Autodesk Fusion 360 part; units mm, degrees
note: some values were not read from the file. Set by a fixed rule: which sketch regions a step uses.
(part 5 of 59)
  spline S22 degree 5 poles (22.1904, 31.2406) (22.1905, 31.2407) (22.1907, 31.2408) (22.1909, 31.241) (22.1913, 31.2414) (22.1919, 31.2419) (22.1925, 31.2424) (22.1933, 31.2431) (22.1941, 31.2438) (22.195, 31.2446) (22.196, 31.2455) (22.197, 31.2464) (22.1982, 31.2474) (22.1994, 31.2485) (22.2007, 31.2497) (22.202, 31.2509) (22.2035, 31.2522) (22.205, 31.2536) (22.2066, 31.255) (22.2082, 31.2565) (22.2099, 31.2581) (22.2117, 31.2597) (22.2136, 31.2615) (22.2155, 31.2632) (22.2175, 31.2651) (22.2195, 31.267) (22.2216, 31.269) (22.2238, 31.271) (22.226, 31.2732) (22.2283, 31.2753) (22.2307, 31.2776) (22.2331, 31.2799) (22.2355, 31.2823) (22.238, 31.2847) (22.2406, 31.2872) (22.2433, 31.2897) (22.2459, 31.2924) (22.2487, 31.2951) (22.2515, 31.2978) (22.2543, 31.3006) (22.2572, 31.3035) (22.2602, 31.3064) (22.2632, 31.3094) (22.2662, 31.3124) (22.2693, 31.3156) (22.2725, 31.3187) (22.2757, 31.322) (22.2789, 31.3252) (22.2822, 31.3286) (22.2855, 31.332) (22.2889, 31.3355) (22.2923, 31.339) (22.2958, 31.3426) (22.2993, 31.3462) (22.3029, 31.3499) (22.3065, 31.3536) (22.3101, 31.3574) (22.3138, 31.3613) (22.3175, 31.3652) (22.3212, 31.3692) (22.325, 31.3732) (22.3289, 31.3773) (22.3328, 31.3814) (22.3367, 31.3856) (22.3406, 31.3899) (22.3446, 31.3942) (22.3486, 31.3986) (22.3527, 31.403) (22.3568, 31.4074) (22.3609, 31.4119) (22.3651, 31.4165) (22.3693, 31.4211) (22.3736, 31.4258) (22.3778, 31.4306) (22.3821, 31.4353) (22.3865, 31.4402) (22.3909, 31.4451) (22.3953, 31.45) (22.3997, 31.455) (22.4042, 31.46) (22.4087, 31.4651) (22.4132, 31.4703) (22.4177, 31.4755) (22.4223, 31.4807) (22.427, 31.486) (22.4316, 31.4914) (22.4363, 31.4968) (22.441, 31.5022) (22.4457, 31.5077) (22.4505, 31.5133) (22.4553, 31.5189) (22.4601, 31.5246) (22.4649, 31.5303) (22.4698, 31.536) (22.4747, 31.5418) (22.4796, 31.5477) (22.4846, 31.5536) (22.4895, 31.5595) (22.4945, 31.5655) (22.4996, 31.5715) (22.5046, 31.5776) (22.5097, 31.5838) (22.5148, 31.59) (22.5199, 31.5962) (22.525, 31.6025) (22.5302, 31.6088) (22.5354, 31.6152) (22.5406, 31.6216) (22.5458, 31.6281) (22.5511, 31.6346) (22.5564, 31.6412) (22.5617, 31.6478) (22.567, 31.6544) (22.5723, 31.6611) (22.5777, 31.6679) (22.583, 31.6747) (22.5884, 31.6815) (22.5939, 31.6884) (22.5993, 31.6954) (22.6048, 31.7024) (22.6102, 31.7094) (22.6157, 31.7165) (22.6212, 31.7236) (22.6268, 31.7307) (22.6323, 31.7379) (22.6379, 31.7452) (22.6435, 31.7525) (22.6491, 31.7598) (22.6547, 31.7672) (22.6603, 31.7747) (22.666, 31.7821) (22.6716, 31.7897) (22.6773, 31.7972) (22.683, 31.8048) (22.6887, 31.8125) (22.6945, 31.8202) (22.7002, 31.8279) (22.706, 31.8357) (22.7118, 31.8436) (22.7175, 31.8514) (22.7233, 31.8593) (22.7292, 31.8673) (22.735, 31.8753) (22.7408, 31.8834) (22.7467, 31.8914) (22.7526, 31.8996) (22.7585, 31.9078) (22.7644, 31.916) (22.7703, 31.9242) (22.7762, 31.9325) (22.7822, 31.9409) (22.7881, 31.9493) (22.7941, 31.9577) (22.8, 31.9662) (22.806, 31.9747) (22.812, 31.9832) (22.818, 31.9918) (22.8241, 32.0005) (22.8301, 32.0091) (22.8361, 32.0179) (22.8422, 32.0266) (22.8483, 32.0354) (22.8543, 32.0443) (22.8604, 32.0532) (22.8665, 32.0621) (22.8726, 32.0711) (22.8787, 32.0801) (22.8849, 32.0891) (22.891, 32.0982) (22.8971, 32.1073) (22.9033, 32.1165) (22.9095, 32.1257) (22.9156, 32.135) (22.9218, 32.1443) (22.928, 32.1536) (22.9342, 32.163) (22.9404, 32.1724) (22.9466, 32.1818) (22.9528, 32.1913) (22.9591, 32.2009) (22.9653, 32.2104) (22.9715, 32.22) (22.9778, 32.2297) (22.984, 32.2394) (22.9903, 32.2491) (22.9966, 32.2589) (23.0029, 32.2687) (23.0091, 32.2785) (23.0154, 32.2884) (23.0217, 32.2984) (23.028, 32.3083) (23.0343, 32.3183) (23.0406, 32.3284) (23.047, 32.3384) (23.0533, 32.3486) (23.0596, 32.3587) (23.066, 32.3689) (23.0723, 32.3791) (23.0786, 32.3894) (23.085, 32.3997) (23.0914, 32.4101) (23.0977, 32.4205) (23.1041, 32.4309) (23.1104, 32.4413) (23.1168, 32.4518) (23.1232, 32.4624) (23.1296, 32.473) (23.136, 32.4836) (23.1423, 32.4942) (23.1487, 32.5049) (23.1551, 32.5156) (23.1615, 32.5264) (23.1679, 32.5372) (23.1743, 32.548) (23.1807, 32.5589) (23.1872, 32.5698) (23.1936, 32.5808) (23.2, 32.5917) (23.2064, 32.6028) (23.2128, 32.6138) (23.2193, 32.6249) (23.2257, 32.636) (23.2321, 32.6472) (23.2385, 32.6584) (23.245, 32.6697) (23.2514, 32.6809) (23.2578, 32.6922) (23.2643, 32.7036) (23.2707, 32.715) (23.2771, 32.7264) (23.2836, 32.7379) (23.29, 32.7493) (23.2965, 32.7609) (23.3029, 32.7724) (23.3094, 32.784) (23.3158, 32.7957) (23.3222, 32.8073) (23.3287, 32.819) (23.3351, 32.8308) (23.3416, 32.8426) (23.348, 32.8544) (23.3532, 32.8639) (23.3571, 32.871) (23.3596, 32.8757) (23.3609, 32.8781) knots 0 0 0 0 0 0 0.00416667 0.00833333 0.0125 0.01666667 0.02083333 0.025 0.02916667 0.03333333 0.0375 0.04166667 0.04583333 0.05 0.05416667 0.05833333 0.0625 0.06666667 0.07083333 0.075 0.07916667 0.08333333 0.0875 0.09166667 0.09583333 0.1 0.10416667 0.10833333 0.1125 0.11666667 0.12083333 0.125 0.12916667 0.13333333 0.1375 0.14166667 0.14583333 0.15 0.15416667 0.15833333 0.1625 0.16666667 0.17083333 0.175 0.17916667 0.18333333 0.1875 0.19166667 0.19583333 0.2 0.20416667 0.20833333 0.2125 0.21666667 0.22083333 0.225 0.22916667 0.23333333 0.2375 0.24166667 0.24583333 0.25 0.25416667 0.25833333 0.2625 0.26666667 0.27083333 0.275 0.27916667 0.28333333 0.2875 0.29166667 0.29583333 0.3 0.30416667 0.30833333 0.3125 0.31666667 0.32083333 0.325 0.32916667 0.33333333 0.3375 0.34166667 0.34583333 0.35 0.35416667 0.35833333 0.3625 0.36666667 0.37083333 0.375 0.37916667 0.38333333 0.3875 0.39166667 0.39583333 0.4 0.40416667 0.40833333 0.4125 0.41666667 0.42083333 0.425 0.42916667 0.43333333 0.4375 0.44166667 0.44583333 0.45 0.45416667 0.45833333 0.4625 0.46666667 0.47083333 0.475 0.47916667 0.48333333 0.4875 0.49166667 0.49583333 0.5 0.50416667 0.50833333 0.5125 0.51666667 0.52083333 0.525 0.52916667 0.53333333 0.5375 0.54166667 0.54583333 0.55 0.55416667 0.55833333 0.5625 0.56666667 0.57083333 0.575 0.57916667 0.58333333 0.5875 0.59166667 0.59583333 0.6 0.60416667 0.60833333 0.6125 0.61666667 0.62083333 0.625 0.62916667 0.63333333 0.6375 0.64166667 0.64583333 0.65 0.65416667 0.65833333 0.6625 0.66666667 0.67083333 0.675 0.67916667 0.68333333 0.6875 0.69166667 0.69583333 0.7 0.70416667 0.70833333 0.7125 0.71666667 0.72083333 0.725 0.72916667 0.73333333 0.7375 0.74166667 0.74583333 0.75 0.75416667 0.75833333 0.7625 0.76666667 0.77083333 0.775 0.77916667 0.78333333 0.7875 0.79166667 0.79583333 0.8 0.80416667 0.80833333 0.8125 0.81666667 0.82083333 0.825 0.82916667 0.83333333 0.8375 0.84166667 0.84583333 0.85 0.85416667 0.85833333 0.8625 0.86666667 0.87083333 0.875 0.87916667 0.88333333 0.8875 0.89166667 0.89583333 0.9 0.90416667 0.90833333 0.9125 0.91666667 0.92083333 0.925 0.92916667 0.93333333 0.9375 0.94166667 0.94583333 0.95 0.95416667 0.95833333 0.9625 0.96666667 0.97083333 0.975 0.97916667 0.98333333 0.9875 0.99166667 0.99583333 1 1 1 1 1 1
  line L72 (-28.5878, 17.6346) -> (-28.587, 17.6345)
  line L73 (-15.1575, -11.9297) -> (-15.3128, -12.1799)
  line L74 (-27.918, 19.3665) -> (-28.2039, 19.4368)
  spline S23 degree 5 poles (-29.3284, 2.4579) (-29.3257, 2.4578) (-29.3203, 2.4577) (-29.3122, 2.4575) (-29.3014, 2.4572) (-29.288, 2.4569) (-29.2745, 2.4566) (-29.2612, 2.4563) (-29.2478, 2.456) (-29.2345, 2.4558) (-29.2212, 2.4555) (-29.2079, 2.4553) (-29.1947, 2.4551) (-29.1815, 2.4549) (-29.1683, 2.4547) (-29.1551, 2.4546) (-29.142, 2.4545) (-29.129, 2.4543) (-29.1159, 2.4542) (-29.1029, 2.4542) (-29.0899, 2.4541) (-29.077, 2.454) (-29.0641, 2.454) (-29.0512, 2.454) (-29.0383, 2.454) (-29.0255, 2.454) (-29.0127, 2.454) (-29, 2.4541) (-28.9872, 2.4542) (-28.9745, 2.4542) (-28.9619, 2.4543) (-28.9493, 2.4544) (-28.9367, 2.4546) (-28.9241, 2.4547) (-28.9116, 2.4549) (-28.8991, 2.4551) (-28.8867, 2.4552) (-28.8743, 2.4555) (-28.8619, 2.4557) (-28.8495, 2.4559) (-28.8372, 2.4562) (-28.8249, 2.4564) (-28.8127, 2.4567) (-28.8005, 2.457) (-28.7883, 2.4573) (-28.7762, 2.4577) (-28.7641, 2.458) (-28.752, 2.4584) (-28.74, 2.4588) (-28.728, 2.4591) (-28.716, 2.4595) (-28.7041, 2.46) (-28.6922, 2.4604) (-28.6803, 2.4608) (-28.6685, 2.4613) (-28.6567, 2.4618) (-28.645, 2.4623) (-28.6333, 2.4628) (-28.6216, 2.4633) (-28.61, 2.4638) (-28.5984, 2.4644) (-28.5868, 2.4649) (-28.5753, 2.4655) (-28.5638, 2.4661) (-28.5524, 2.4667) (-28.541, 2.4673) (-28.5296, 2.4679) (-28.5183, 2.4686) (-28.507, 2.4692) (-28.4957, 2.4699) (-28.4845, 2.4706) (-28.4733, 2.4713) (-28.4622, 2.472) (-28.4511, 2.4727) (-28.44, 2.4734) (-28.429, 2.4742) (-28.4181, 2.4749) (-28.4071, 2.4757) (-28.3962, 2.4765) (-28.3854, 2.4773) (-28.3745, 2.4781) (-28.3638, 2.4789) (-28.353, 2.4797) (-28.3423, 2.4805) (-28.3317, 2.4814) (-28.321, 2.4823) (-28.3105, 2.4831) (-28.2999, 2.484) (-28.2894, 2.4849) (-28.279, 2.4858) (-28.2686, 2.4867) (-28.2582, 2.4877) (-28.2479, 2.4886) (-28.2376, 2.4896) (-28.2274, 2.4905) (-28.2172, 2.4915) (-28.207, 2.4925) (-28.1969, 2.4935) (-28.1868, 2.4945) (-28.1768, 2.4955) (-28.1668, 2.4965) (-28.1569, 2.4975) (-28.147, 2.4986) (-28.1372, 2.4996) (-28.1274, 2.5007) (-28.1176, 2.5017) (-28.1079, 2.5028) (-28.0982, 2.5039) (-28.0886, 2.505) (-28.079, 2.5061) (-28.0695, 2.5072) (-28.06, 2.5084) (-28.0506, 2.5095) (-28.0412, 2.5106) (-28.0318, 2.5118) (-28.0225, 2.5129) (-28.0133, 2.5141) (-28.004, 2.5153) (-27.9949, 2.5164) (-27.9858, 2.5176) (-27.9767, 2.5188) (-27.9677, 2.52) (-27.9587, 2.5212) (-27.9498, 2.5224) (-27.9409, 2.5237) (-27.9321, 2.5249) (-27.9233, 2.5261) (-27.9146, 2.5274) (-27.9059, 2.5286) (-27.8973, 2.5299) (-27.8887, 2.5311) (-27.8802, 2.5324) (-27.8717, 2.5336) (-27.8633, 2.5349) (-27.8549, 2.5362) (-27.8466, 2.5375) (-27.8383, 2.5388) (-27.8301, 2.5401) (-27.8219, 2.5414) (-27.8138, 2.5427) (-27.8057, 2.544) (-27.7977, 2.5453) (-27.7898, 2.5466) (-27.7819, 2.5479) (-27.774, 2.5492) (-27.7662, 2.5506) (-27.7585, 2.5519) (-27.7508, 2.5532) (-27.7431, 2.5546) (-27.7356, 2.5559) (-27.728, 2.5572) (-27.7206, 2.5586) (-27.7132, 2.5599) (-27.7058, 2.5613) (-27.6985, 2.5626) (-27.6912, 2.564) (-27.6841, 2.5653) (-27.6769, 2.5667) (-27.6698, 2.568) (-27.6628, 2.5694) (-27.6559, 2.5707) (-27.649, 2.5721) (-27.6421, 2.5734) (-27.6353, 2.5748) (-27.6286, 2.5761) (-27.622, 2.5775) (-27.6154, 2.5788) (-27.6088, 2.5801) (-27.6023, 2.5815) (-27.5959, 2.5828) (-27.5896, 2.5842) (-27.5833, 2.5855) (-27.577, 2.5868) (-27.5709, 2.5882) (-27.5647, 2.5895) (-27.5587, 2.5908) (-27.5527, 2.5921) (-27.5468, 2.5935) (-27.5409, 2.5948) (-27.5352, 2.5961) (-27.5294, 2.5974) (-27.5238, 2.5987) (-27.5182, 2.6) (-27.5127, 2.6013) (-27.5072, 2.6026) (-27.5018, 2.6038) (-27.4965, 2.6051) (-27.4912, 2.6064) (-27.4861, 2.6076) (-27.481, 2.6089) (-27.4759, 2.6101) (-27.4709, 2.6113) (-27.466, 2.6126) (-27.4612, 2.6138) (-27.4564, 2.615) (-27.4517, 2.6162) (-27.4471, 2.6173) (-27.4426, 2.6185) (-27.4381, 2.6197) (-27.4337, 2.6208) (-27.4294, 2.622) (-27.4252, 2.6231) (-27.421, 2.6242) (-27.4169, 2.6253) (-27.4129, 2.6264) (-27.409, 2.6275) (-27.4051, 2.6285) (-27.4013, 2.6296) (-27.3976, 2.6306) (-27.394, 2.6316) (-27.3905, 2.6326) (-27.387, 2.6336) (-27.3837, 2.6346) (-27.3804, 2.6355) (-27.3772, 2.6365) (-27.3741, 2.6374) (-27.371, 2.6383) (-27.3681, 2.6392) (-27.3652, 2.64) (-27.3625, 2.6409) (-27.3598, 2.6417) (-27.3572, 2.6425) (-27.3547, 2.6432) (-27.3523, 2.644) (-27.3499, 2.6447) (-27.3477, 2.6454) (-27.3456, 2.6461) (-27.3435, 2.6467) (-27.3416, 2.6473) (-27.3398, 2.6479) (-27.338, 2.6485) (-27.3364, 2.649) (-27.3348, 2.6495) (-27.3334, 2.65) (-27.332, 2.6505) (-27.3308, 2.6509) (-27.3296, 2.6513) (-27.3286, 2.6516) (-27.3277, 2.6519) (-27.3269, 2.6522) (-27.3262, 2.6525) (-27.3257, 2.6526) (-27.3254, 2.6527) (-27.3252, 2.6528) (-27.3251, 2.6528) knots -1 -1 -1 -1 -1 -1 -0.99583333 -0.99166667 -0.9875 -0.98333333 -0.97916667 -0.975 -0.97083333 -0.96666667 -0.9625 -0.95833333 -0.95416667 -0.95 -0.94583333 -0.94166667 -0.9375 -0.93333333 -0.92916667 -0.925 -0.92083333 -0.91666667 -0.9125 -0.90833333 -0.90416667 -0.9 -0.89583333 -0.89166667 -0.8875 -0.88333333 -0.87916667 -0.875 -0.87083333 -0.86666667 -0.8625 -0.85833333 -0.85416667 -0.85 -0.84583333 -0.84166667 -0.8375 -0.83333333 -0.82916667 -0.825 -0.82083333 -0.81666667 -0.8125 -0.80833333 -0.80416667 -0.8 -0.79583333 -0.79166667 -0.7875 -0.78333333 -0.77916667 -0.775 -0.77083333 -0.76666667 -0.7625 -0.75833333 -0.75416667 -0.75 -0.74583333 -0.74166667 -0.7375 -0.73333333 -0.72916667 -0.725 -0.72083333 -0.71666667 -0.7125 -0.70833333 -0.70416667 -0.7 -0.69583333 -0.69166667 -0.6875 -0.68333333 -0.67916667 -0.675 -0.67083333 -0.66666667 -0.6625 -0.65833333 -0.65416667 -0.65 -0.64583333 -0.64166667 -0.6375 -0.63333333 -0.62916667 -0.625 -0.62083333 -0.61666667 -0.6125 -0.60833333 -0.60416667 -0.6 -0.59583333 -0.59166667 -0.5875 -0.58333333 -0.57916667 -0.575 -0.57083333 -0.56666667 -0.5625 -0.55833333 -0.55416667 -0.55 -0.54583333 -0.54166667 -0.5375 -0.53333333 -0.52916667 -0.525 -0.52083333 -0.51666667 -0.5125 -0.50833333 -0.50416667 -0.5 -0.49583333 -0.49166667 -0.4875 -0.48333333 -0.47916667 -0.475 -0.47083333 -0.46666667 -0.4625 -0.45833333 -0.45416667 -0.45 -0.44583333 -0.44166667 -0.4375 -0.43333333 -0.42916667 -0.425 -0.42083333 -0.41666667 -0.4125 -0.40833333 -0.40416667 -0.4 -0.39583333 -0.39166667 -0.3875 -0.38333333 -0.37916667 -0.375 -0.37083333 -0.36666667 -0.3625 -0.35833333 -0.35416667 -0.35 -0.34583333 -0.34166667 -0.3375 -0.33333333 -0.32916667 -0.325 -0.32083333 -0.31666667 -0.3125 -0.30833333 -0.30416667 -0.3 -0.29583333 -0.29166667 -0.2875 -0.28333333 -0.27916667 -0.275 -0.27083333 -0.26666667 -0.2625 -0.25833333 -0.25416667 -0.25 -0.24583333 -0.24166667 -0.2375 -0.23333333 -0.22916667 -0.225 -0.22083333 -0.21666667 -0.2125 -0.20833333 -0.20416667 -0.2 -0.19583333 -0.19166667 -0.1875 -0.18333333 -0.17916667 -0.175 -0.17083333 -0.16666667 -0.1625 -0.15833333 -0.15416667 -0.15 -0.14583333 -0.14166667 -0.1375 -0.13333333 -0.12916667 -0.125 -0.12083333 -0.11666667 -0.1125 -0.10833333 -0.10416667 -0.1 -0.09583333 -0.09166667 -0.0875 -0.08333333 -0.07916667 -0.075 -0.07083333 -0.06666667 -0.0625 -0.05833333 -0.05416667 -0.05 -0.04583333 -0.04166667 -0.0375 -0.03333333 -0.02916667 -0.025 -0.02083333 -0.01666667 -0.0125 -0.00833333 -0.00416667 0 0 0 0 0 0
  line L75 (-25.6012, -1.2171) -> (-25.6019, -1.2175)
  line L76 (-26.1461, -0.1495) -> (-26.1453, -0.1491)
  arc A31 (-27.6109, 20.5125) -> (-27.918, 19.3665) centre (0, 12.5) ccw
  arc A32 (-30.2174, 19.4214) -> (-30.4202, 18.4675) centre (0, 12.5) ccw
  spline S24 degree 5 poles (-30.4202, 18.4675) (-30.4179, 18.4661) (-30.4133, 18.4633) (-30.4064, 18.459) (-30.3972, 18.4534) (-30.3857, 18.4464) (-30.3742, 18.4394) (-30.3628, 18.4325) (-30.3513, 18.4255) (-30.3399, 18.4187) (-30.3285, 18.4118) (-30.3171, 18.405) (-30.3058, 18.3982) (-30.2944, 18.3914) (-30.2831, 18.3847) (-30.2718, 18.378) (-30.2605, 18.3713) (-30.2492, 18.3647) (-30.238, 18.3581) (-30.2268, 18.3515) (-30.2156, 18.3449) (-30.2044, 18.3384) (-30.1932, 18.3319) (-30.1821, 18.3255) (-30.1709, 18.3191) (-30.1598, 18.3127) (-30.1487, 18.3063) (-30.1377, 18.3) (-30.1266, 18.2937) (-30.1156, 18.2874) (-30.1046, 18.2811) (-30.0936, 18.2749) (-30.0826, 18.2688) (-30.0717, 18.2626) (-30.0608, 18.2565) (-30.0499, 18.2504) (-30.039, 18.2443) (-30.0281, 18.2383) (-30.0173, 18.2323) (-30.0065, 18.2263) (-29.9957, 18.2204) (-29.9849, 18.2145) (-29.9742, 18.2086) (-29.9634, 18.2028) (-29.9527, 18.197) (-29.9421, 18.1912) (-29.9314, 18.1854) (-29.9208, 18.1797) (-29.9102, 18.174) (-29.8996, 18.1683) (-29.889, 18.1627) (-29.8785, 18.1571) (-29.868, 18.1515) (-29.8575, 18.146) (-29.847, 18.1405) (-29.8366, 18.135) (-29.8262, 18.1296) (-29.8158, 18.1242) (-29.8054, 18.1188) (-29.7951, 18.1134) (-29.7847, 18.1081) (-29.7745, 18.1028) (-29.7642, 18.0975) (-29.754, 18.0923) (-29.7437, 18.0871) (-29.7336, 18.0819) (-29.7234, 18.0768) (-29.7133, 18.0717) (-29.7032, 18.0666) (-29.6931, 18.0615) (-29.683, 18.0565) (-29.673, 18.0515) (-29.663, 18.0466) (-29.653, 18.0416) (-29.6431, 18.0367) (-29.6332, 18.0319) (-29.6233, 18.027) (-29.6134, 18.0222) (-29.6036, 18.0175) (-29.5938, 18.0127) (-29.584, 18.008) (-29.5743, 18.0033) (-29.5646, 17.9987) (-29.5549, 17.994) (-29.5452, 17.9895) (-29.5356, 17.9849) (-29.526, 17.9804) (-29.5165, 17.9759) (-29.5069, 17.9714) (-29.4974, 17.967) (-29.4879, 17.9625) (-29.4785, 17.9582) (-29.4691, 17.9538) (-29.4597, 17.9495) (-29.4504, 17.9452) (-29.441, 17.941) (-29.4318, 17.9367) (-29.4225, 17.9325) (-29.4133, 17.9284) (-29.4041, 17.9242) (-29.395, 17.9201) (-29.3858, 17.9161) (-29.3767, 17.912) (-29.3677, 17.908) (-29.3587, 17.904) (-29.3497, 17.9001) (-29.3407, 17.8961) (-29.3318, 17.8922) (-29.3229, 17.8884) (-29.3141, 17.8846) (-29.3053, 17.8807) (-29.2965, 17.877) (-29.2878, 17.8732) (-29.279, 17.8695) (-29.2704, 17.8658) (-29.2617, 17.8622) (-29.2531, 17.8586) (-29.2446, 17.855) (-29.2361, 17.8514) (-29.2276, 17.8479) (-29.2191, 17.8444) (-29.2107, 17.8409) (-29.2023, 17.8375) (-29.194, 17.8341) (-29.1857, 17.8307) (-29.1775, 17.8273) (-29.1692, 17.824) (-29.1611, 17.8207) (-29.1529, 17.8175) (-29.1448, 17.8143) (-29.1368, 17.8111) (-29.1288, 17.8079) (-29.1208, 17.8047) (-29.1129, 17.8016) (-29.105, 17.7986) (-29.0971, 17.7955) (-29.0893, 17.7925) (-29.0815, 17.7895) (-29.0738, 17.7865) (-29.0661, 17.7836) (-29.0585, 17.7807) (-29.0509, 17.7778) (-29.0433, 17.775) (-29.0358, 17.7722) (-29.0284, 17.7694) (-29.021, 17.7666) (-29.0136, 17.7639) (-29.0063, 17.7612) (-28.999, 17.7586) (-28.9918, 17.7559) (-28.9846, 17.7533) (-28.9774, 17.7508) (-28.9703, 17.7482) (-28.9633, 17.7457) (-28.9563, 17.7432) (-28.9493, 17.7408) (-28.9424, 17.7383) (-28.9356, 17.7359) (-28.9288, 17.7336) (-28.922, 17.7312) (-28.9153, 17.7289) (-28.9087, 17.7266) (-28.9021, 17.7244) (-28.8955, 17.7222) (-28.889, 17.72) (-28.8826, 17.7178) (-28.8762, 17.7157) (-28.8699, 17.7136) (-28.8636, 17.7115) (-28.8573, 17.7094) (-28.8512, 17.7074) (-28.8451, 17.7054) (-28.839, 17.7035) (-28.833, 17.7015) (-28.827, 17.6996) (-28.8211, 17.6978) (-28.8153, 17.6959) (-28.8095, 17.6941) (-28.8038, 17.6923) (-28.7981, 17.6905) (-28.7925, 17.6888) (-28.7869, 17.6871) (-28.7815, 17.6854) (-28.776, 17.6838) (-28.7707, 17.6822) (-28.7654, 17.6806) (-28.7601, 17.679) (-28.7549, 17.6775) (-28.7498, 17.676) (-28.7448, 17.6745) (-28.7398, 17.673) (-28.7349, 17.6716) (-28.73, 17.6702) (-28.7252, 17.6689) (-28.7205, 17.6675) (-28.7158, 17.6662) (-28.7112, 17.6649) (-28.7067, 17.6637) (-28.7023, 17.6625) (-28.6979, 17.6613) (-28.6936, 17.6601) (-28.6893, 17.6589) (-28.6852, 17.6578) (-28.6811, 17.6567) (-28.6771, 17.6557) (-28.6731, 17.6546) (-28.6693, 17.6536) (-28.6655, 17.6527) (-28.6617, 17.6517) (-28.6581, 17.6508) (-28.6545, 17.6499) (-28.6511, 17.649) (-28.6477, 17.6481) (-28.6443, 17.6473) (-28.6411, 17.6465) (-28.6379, 17.6458) (-28.6349, 17.645) (-28.6319, 17.6443) (-28.629, 17.6436) (-28.6262, 17.643) (-28.6234, 17.6423) (-28.6208, 17.6417) (-28.6182, 17.6411) (-28.6158, 17.6406) (-28.6134, 17.64) (-28.6111, 17.6395) (-28.6089, 17.639) (-28.6069, 17.6386) (-28.6049, 17.6381) (-28.603, 17.6377) (-28.6012, 17.6374) (-28.5995, 17.637) (-28.5979, 17.6367) (-28.5964, 17.6363) (-28.595, 17.6361) (-28.5937, 17.6358) (-28.5925, 17.6356) (-28.5915, 17.6354) (-28.5905, 17.6352) (-28.5896, 17.635) (-28.5889, 17.6349) (-28.5884, 17.6348) (-28.5881, 17.6347) (-28.5879, 17.6347) (-28.5878, 17.6346) knots -1 -1 -1 -1 -1 -1 -0.99583333 -0.99166667 -0.9875 -0.98333333 -0.97916667 -0.975 -0.97083333 -0.96666667 -0.9625 -0.95833333 -0.95416667 -0.95 -0.94583333 -0.94166667 -0.9375 -0.93333333 -0.92916667 -0.925 -0.92083333 -0.91666667 -0.9125 -0.90833333 -0.90416667 -0.9 -0.89583333 -0.89166667 -0.8875 -0.88333333 -0.87916667 -0.875 -0.87083333 -0.86666667 -0.8625 -0.85833333 -0.85416667 -0.85 -0.84583333 -0.84166667 -0.8375 -0.83333333 -0.82916667 -0.825 -0.82083333 -0.81666667 -0.8125 -0.80833333 -0.80416667 -0.8 -0.79583333 -0.79166667 -0.7875 -0.78333333 -0.77916667 -0.775 -0.77083333 -0.76666667 -0.7625 -0.75833333 -0.75416667 -0.75 -0.74583333 -0.74166667 -0.7375 -0.73333333 -0.72916667 -0.725 -0.72083333 -0.71666667 -0.7125 -0.70833333 -0.70416667 -0.7 -0.69583333 -0.69166667 -0.6875 -0.68333333 -0.67916667 -0.675 -0.67083333 -0.66666667 -0.6625 -0.65833333 -0.65416667 -0.65 -0.64583333 -0.64166667 -0.6375 -0.63333333 -0.62916667 -0.625 -0.62083333 -0.61666667 -0.6125 -0.60833333 -0.60416667 -0.6 -0.59583333 -0.59166667 -0.5875 -0.58333333 -0.57916667 -0.575 -0.57083333 -0.56666667 -0.5625 -0.55833333 -0.55416667 -0.55 -0.54583333 -0.54166667 -0.5375 -0.53333333 -0.52916667 -0.525 -0.52083333 -0.51666667 -0.5125 -0.50833333 -0.50416667 -0.5 -0.49583333 -0.49166667 -0.4875 -0.48333333 -0.47916667 -0.475 -0.47083333 -0.46666667 -0.4625 -0.45833333 -0.45416667 -0.45 -0.44583333 -0.44166667 -0.4375 -0.43333333 -0.42916667 -0.425 -0.42083333 -0.41666667 -0.4125 -0.40833333 -0.40416667 -0.4 -0.39583333 -0.39166667 -0.3875 -0.38333333 -0.37916667 -0.375 -0.37083333 -0.36666667 -0.3625 -0.35833333 -0.35416667 -0.35 -0.34583333 -0.34166667 -0.3375 -0.33333333 -0.32916667 -0.325 -0.32083333 -0.31666667 -0.3125 -0.30833333 -0.30416667 -0.3 -0.29583333 -0.29166667 -0.2875 -0.28333333 -0.27916667 -0.275 -0.27083333 -0.26666667 -0.2625 -0.25833333 -0.25416667 -0.25 -0.24583333 -0.24166667 -0.2375 -0.23333333 -0.22916667 -0.225 -0.22083333 -0.21666667 -0.2125 -0.20833333 -0.20416667 -0.2 -0.19583333 -0.19166667 -0.1875 -0.18333333 -0.17916667 -0.175 -0.17083333 -0.16666667 -0.1625 -0.15833333 -0.15416667 -0.15 -0.14583333 -0.14166667 -0.1375 -0.13333333 -0.12916667 -0.125 -0.12083333 -0.11666667 -0.1125 -0.10833333 -0.10416667 -0.1 -0.09583333 -0.09166667 -0.0875 -0.08333333 -0.07916667 -0.075 -0.07083333 -0.06666667 -0.0625 -0.05833333 -0.05416667 -0.05 -0.04583333 -0.04166667 -0.0375 -0.03333333 -0.02916667 -0.025 -0.02083333 -0.01666667 -0.0125 -0.00833333 -0.00416667 0 0 0 0 0 0
  arc A33 (-28.2972, 17.5824) -> (-28.4828, 16.4106) centre (0, 12.5) ccw
  line L77 (-28.7753, 8.5492) -> (-28.7745, 8.5493)
  arc A34 (-28.5147, 0.3382) -> (-28.1181, -0.5527) centre (0, 12.5) ccw
  line L78 (-24.6799, -2.8128) -> (-24.4297, -2.6575)
  line L79 (-28.7745, 8.5493) -> (-28.4828, 8.5894)
  line L80 (-29.0307, 11.5787) -> (-29.0298, 11.5787)
  line L81 (-21.9649, -6.0501) -> (-22.1898, -6.2401)
  line L82 (-28.9671, 10.3818) -> (-28.9679, 10.3817)
  arc A35 (-27.0873, -2.5758) -> (-26.5997, -3.4204) centre (0, 12.5) ccw
  spline S25 degree 5 poles (-15.3132, -12.1806) (-15.3132, -12.1807) (-15.3133, -12.1809) (-15.3135, -12.1812) (-15.3138, -12.1816) (-15.3142, -12.1822) (-15.3146, -12.183) (-15.3151, -12.1838) (-15.3157, -12.1848) (-15.3163, -12.1858) (-15.3169, -12.1869) (-15.3177, -12.1881) (-15.3184, -12.1895) (-15.3193, -12.1909) (-15.3201, -12.1924) (-15.321, -12.194) (-15.322, -12.1956) (-15.323, -12.1974) (-15.3241, -12.1993) (-15.3252, -12.2012) (-15.3263, -12.2033) (-15.3275, -12.2054) (-15.3287, -12.2076) (-15.33, -12.2099) (-15.3313, -12.2122) (-15.3327, -12.2147) (-15.3341, -12.2172) (-15.3355, -12.2198) (-15.337, -12.2225) (-15.3385, -12.2253) (-15.34, -12.2282) (-15.3416, -12.2311) (-15.3432, -12.2341) (-15.3449, -12.2372) (-15.3465, -12.2404) (-15.3482, -12.2437) (-15.35, -12.247) (-15.3518, -12.2504) (-15.3536, -12.2539) (-15.3554, -12.2574) (-15.3573, -12.261) (-15.3592, -12.2647) (-15.3611, -12.2685) (-15.3631, -12.2723) (-15.3651, -12.2763) (-15.3671, -12.2802) (-15.3691, -12.2843) (-15.3712, -12.2884) (-15.3733, -12.2926) (-15.3754, -12.2969) (-15.3775, -12.3012) (-15.3797, -12.3056) (-15.3819, -12.3101) (-15.3841, -12.3147) (-15.3863, -12.3193) (-15.3886, -12.3239) (-15.3909, -12.3287) (-15.3932, -12.3335) (-15.3955, -12.3384) (-15.3979, -12.3433) (-15.4002, -12.3483) (-15.4026, -12.3534) (-15.405, -12.3585) (-15.4075, -12.3637) (-15.4099, -12.369) (-15.4124, -12.3743) (-15.4149, -12.3797) (-15.4174, -12.3852) (-15.4199, -12.3907) (-15.4224, -12.3962) (-15.425, -12.4019) (-15.4275, -12.4076) (-15.4301, -12.4133) (-15.4327, -12.4192) (-15.4353, -12.425) (-15.438, -12.431) (-15.4406, -12.437) (-15.4433, -12.443) (-15.446, -12.4492) (-15.4486, -12.4553) (-15.4514, -12.4616) (-15.4541, -12.4679) (-15.4568, -12.4742) (-15.4595, -12.4806) (-15.4623, -12.4871) (-15.4651, -12.4936) (-15.4678, -12.5002) (-15.4706, -12.5069) (-15.4734, -12.5136) (-15.4762, -12.5203) (-15.4791, -12.5271) (-15.4819, -12.534) (-15.4848, -12.5409) (-15.4876, -12.5479) (-15.4905, -12.5549) (-15.4933, -12.562) (-15.4962, -12.5691) (-15.4991, -12.5763) (-15.502, -12.5836) (-15.5049, -12.5909) (-15.5078, -12.5982) (-15.5108, -12.6056) (-15.5137, -12.6131) (-15.5166, -12.6206) (-15.5196, -12.6282) (-15.5226, -12.6358) (-15.5255, -12.6434) (-15.5285, -12.6512) (-15.5315, -12.6589) (-15.5344, -12.6668) (-15.5374, -12.6746) (-15.5404, -12.6826) (-15.5434, -12.6905) (-15.5464, -12.6986) (-15.5494, -12.7066) (-15.5524, -12.7148) (-15.5555, -12.7229) (-15.5585, -12.7312) (-15.5615, -12.7394) (-15.5645, -12.7478) (-15.5676, -12.7562) (-15.5706, -12.7646) (-15.5737, -12.7731) (-15.5767, -12.7816) (-15.5798, -12.7901) (-15.5828, -12.7988) (-15.5859, -12.8074) (-15.5889, -12.8161) (-15.592, -12.8249) (-15.595, -12.8337) (-15.5981, -12.8426) (-15.6012, -12.8515) (-15.6042, -12.8604) (-15.6073, -12.8694) (-15.6104, -12.8785) (-15.6134, -12.8876) (-15.6165, -12.8967) (-15.6196, -12.9059) (-15.6227, -12.9151) (-15.6257, -12.9244) (-15.6288, -12.9337) (-15.6319, -12.9431) (-15.635, -12.9525) (-15.638, -12.962) (-15.6411, -12.9715) (-15.6442, -12.981) (-15.6473, -12.9906) (-15.6503, -13.0003) (-15.6534, -13.0099) (-15.6565, -13.0197) (-15.6596, -13.0294) (-15.6626, -13.0393) (-15.6657, -13.0491) (-15.6688, -13.059) (-15.6718, -13.069) (-15.6749, -13.079) (-15.6779, -13.089) (-15.681, -13.0991) (-15.6841, -13.1092) (-15.6871, -13.1194) (-15.6902, -13.1296) (-15.6932, -13.1398) (-15.6963, -13.1501) (-15.6993, -13.1604) (-15.7023, -13.1708) (-15.7054, -13.1812) (-15.7084, -13.1917) (-15.7114, -13.2022) (-15.7145, -13.2127) (-15.7175, -13.2233) (-15.7205, -13.2339) (-15.7235, -13.2446) (-15.7265, -13.2553) (-15.7295, -13.266) (-15.7325, -13.2768) (-15.7355, -13.2877) (-15.7385, -13.2985) (-15.7415, -13.3094) (-15.7445, -13.3204) (-15.7475, -13.3314) (-15.7504, -13.3424) (-15.7534, -13.3535) (-15.7564, -13.3646) (-15.7593, -13.3757) (-15.7623, -13.3869) (-15.7652, -13.3982) (-15.7682, -13.4094) (-15.7711, -13.4207) (-15.774, -13.4321) (-15.7769, -13.4435) (-15.7798, -13.4549) (-15.7828, -13.4663) (-15.7857, -13.4778) (-15.7886, -13.4894) (-15.7914, -13.501) (-15.7943, -13.5126) (-15.7972, -13.5242) (-15.8001, -13.5359) (-15.8029, -13.5477) (-15.8058, -13.5594) (-15.8086, -13.5712) (-15.8115, -13.5831) (-15.8143, -13.595) (-15.8171, -13.6069) (-15.8199, -13.6188) (-15.8227, -13.6308) (-15.8255, -13.6428) (-15.8283, -13.6549) (-15.8311, -13.667) (-15.8339, -13.6792) (-15.8367, -13.6913) (-15.8394, -13.7035) (-15.8422, -13.7158) (-15.8449, -13.7281) (-15.8477, -13.7404) (-15.8504, -13.7528) (-15.8531, -13.7651) (-15.8558, -13.7776) (-15.8585, -13.79) (-15.8612, -13.8025) (-15.8639, -13.8151) (-15.8666, -13.8276) (-15.8692, -13.8403) (-15.8719, -13.8529) (-15.8745, -13.8656) (-15.8771, -13.8783) (-15.8798, -13.891) (-15.8824, -13.9038) (-15.885, -13.9166) (-15.8876, -13.9295) (-15.8902, -13.9424) (-15.8927, -13.9553) (-15.8953, -13.9682) (-15.8979, -13.9812) (-15.9004, -13.9943) (-15.9029, -14.0073) (-15.9055, -14.0204) (-15.908, -14.0335) (-15.9105, -14.0467) (-15.913, -14.0599) (-15.9154, -14.0731) (-15.9174, -14.0837) (-15.9189, -14.0917) (-15.9199, -14.097) (-15.9204, -14.0997) knots 0 0 0 0 0 0 0.00416667 0.00833333 0.0125 0.01666667 0.02083333 0.025 0.02916667 0.03333333 0.0375 0.04166667 0.04583333 0.05 0.05416667 0.05833333 0.0625 0.06666667 0.07083333 0.075 0.07916667 0.08333333 0.0875 0.09166667 0.09583333 0.1 0.10416667 0.10833333 0.1125 0.11666667 0.12083333 0.125 0.12916667 0.13333333 0.1375 0.14166667 0.14583333 0.15 0.15416667 0.15833333 0.1625 0.16666667 0.17083333 0.175 0.17916667 0.18333333 0.1875 0.19166667 0.19583333 0.2 0.20416667 0.20833333 0.2125 0.21666667 0.22083333 0.225 0.22916667 0.23333333 0.2375 0.24166667 0.24583333 0.25 0.25416667 0.25833333 0.2625 0.26666667 0.27083333 0.275 0.27916667 0.28333333 0.2875 0.29166667 0.29583333 0.3 0.30416667 0.30833333 0.3125 0.31666667 0.32083333 0.325 0.32916667 0.33333333 0.3375 0.34166667 0.34583333 0.35 0.35416667 0.35833333 0.3625 0.36666667 0.37083333 0.375 0.37916667 0.38333333 0.3875 0.39166667 0.39583333 0.4 0.40416667 0.40833333 0.4125 0.41666667 0.42083333 0.425 0.42916667 0.43333333 0.4375 0.44166667 0.44583333 0.45 0.45416667 0.45833333 0.4625 0.46666667 0.47083333 0.475 0.47916667 0.48333333 0.4875 0.49166667 0.49583333 0.5 0.50416667 0.50833333 0.5125 0.51666667 0.52083333 0.525 0.52916667 0.53333333 0.5375 0.54166667 0.54583333 0.55 0.55416667 0.55833333 0.5625 0.56666667 0.57083333 0.575 0.57916667 0.58333333 0.5875 0.59166667 0.59583333 0.6 0.60416667 0.60833333 0.6125 0.61666667 0.62083333 0.625 0.62916667 0.63333333 0.6375 0.64166667 0.64583333 0.65 0.65416667 0.65833333 0.6625 0.66666667 0.67083333 0.675 0.67916667 0.68333333 0.6875 0.69166667 0.69583333 0.7 0.70416667 0.70833333 0.7125 0.71666667 0.72083333 0.725 0.72916667 0.73333333 0.7375 0.74166667 0.74583333 0.75 0.75416667 0.75833333 0.7625 0.76666667 0.77083333 0.775 0.77916667 0.78333333 0.7875 0.79166667 0.79583333 0.8 0.80416667 0.80833333 0.8125 0.81666667 0.82083333 0.825 0.82916667 0.83333333 0.8375 0.84166667 0.84583333 0.85 0.85416667 0.85833333 0.8625 0.86666667 0.87083333 0.875 0.87916667 0.88333333 0.8875 0.89166667 0.89583333 0.9 0.90416667 0.90833333 0.9125 0.91666667 0.92083333 0.925 0.92916667 0.93333333 0.9375 0.94166667 0.94583333 0.95 0.95416667 0.95833333 0.9625 0.96666667 0.97083333 0.975 0.97916667 0.98333333 0.9875 0.99166667 0.99583333 1 1 1 1 1 1
  line L83 (-19.9055, -8.2445) -> (-20.1094, -8.4569)
  arc A36 (-22.7115, -5.1281) -> (-21.9649, -6.0501) centre (0, 12.5) ccw
  line L84 (-22.9448, -5.3091) -> (-22.9441, -5.3086)
  spline S26 degree 5 poles (-17.8246, -12.863) (-17.8224, -12.8615) (-17.8179, -12.8584) (-17.8112, -12.8539) (-17.8023, -12.8477) (-17.7913, -12.8401) (-17.7802, -12.8325) (-17.7692, -12.8248) (-17.7583, -12.8172) (-17.7473, -12.8096) (-17.7364, -12.8019) (-17.7256, -12.7943) (-17.7147, -12.7867) (-17.7039, -12.7791) (-17.6932, -12.7715) (-17.6825, -12.7639) (-17.6718, -12.7563) (-17.6611, -12.7487) (-17.6505, -12.7411) (-17.6399, -12.7335) (-17.6294, -12.7259) (-17.6189, -12.7184) (-17.6084, -12.7108) (-17.598, -12.7032) (-17.5876, -12.6957) (-17.5772, -12.6881) (-17.5669, -12.6806) (-17.5566, -12.6731) (-17.5464, -12.6655) (-17.5361, -12.658) (-17.526, -12.6505) (-17.5158, -12.643) (-17.5057, -12.6355) (-17.4956, -12.628) (-17.4856, -12.6205) (-17.4756, -12.613) (-17.4657, -12.6055) (-17.4557, -12.5981) (-17.4458, -12.5906) (-17.436, -12.5832) (-17.4262, -12.5757) (-17.4164, -12.5683) (-17.4067, -12.5609) (-17.397, -12.5534) (-17.3873, -12.546) (-17.3777, -12.5386) (-17.3681, -12.5312) (-17.3585, -12.5238) (-17.349, -12.5165) (-17.3395, -12.5091) (-17.3301, -12.5017) (-17.3207, -12.4944) (-17.3113, -12.4871) (-17.302, -12.4797) (-17.2927, -12.4724) (-17.2835, -12.4651) (-17.2743, -12.4578) (-17.2651, -12.4505) (-17.2559, -12.4432) (-17.2469, -12.436) (-17.2378, -12.4287) (-17.2288, -12.4215) (-17.2198, -12.4142) (-17.2108, -12.407) (-17.2019, -12.3998) (-17.1931, -12.3926) (-17.1842, -12.3854) (-17.1754, -12.3782) (-17.1667, -12.3711) (-17.158, -12.3639) (-17.1493, -12.3568) (-17.1407, -12.3496) (-17.1321, -12.3425) (-17.1235, -12.3354) (-17.115, -12.3283) (-17.1065, -12.3212) (-17.0981, -12.3142) (-17.0897, -12.3071) (-17.0813, -12.3001) (-17.073, -12.2931) (-17.0647, -12.2861) (-17.0565, -12.2791) (-17.0483, -12.2721) (-17.0401, -12.2651) (-17.032, -12.2582) (-17.0239, -12.2512) (-17.0159, -12.2443) (-17.0079, -12.2374) (-16.9999, -12.2305) (-16.992, -12.2236) (-16.9841, -12.2168) (-16.9763, -12.2099) (-16.9685, -12.2031) (-16.9607, -12.1963) (-16.953, -12.1895) (-16.9453, -12.1827) (-16.9377, -12.1759) (-16.9301, -12.1692) (-16.9225, -12.1625) (-16.915, -12.1558) (-16.9075, -12.1491) (-16.9001, -12.1424) (-16.8927, -12.1357) (-16.8854, -12.1291) (-16.8781, -12.1225) (-16.8708, -12.1159) (-16.8636, -12.1093) (-16.8564, -12.1027) (-16.8492, -12.0962) (-16.8421, -12.0897) (-16.8351, -12.0831) (-16.8281, -12.0767) (-16.8211, -12.0702) (-16.8142, -12.0638) (-16.8073, -12.0573) (-16.8004, -12.0509) (-16.7936, -12.0446) (-16.7869, -12.0382) (-16.7801, -12.0319) (-16.7735, -12.0255) (-16.7668, -12.0192) (-16.7602, -12.013) (-16.7537, -12.0067) (-16.7472, -12.0005) (-16.7407, -11.9943) (-16.7343, -11.9881) (-16.7279, -11.982) (-16.7216, -11.9758) (-16.7153, -11.9697) (-16.7091, -11.9636) (-16.7029, -11.9576) (-16.6967, -11.9515) (-16.6906, -11.9455) (-16.6845, -11.9395) (-16.6785, -11.9336) (-16.6725, -11.9277) (-16.6666, -11.9218) (-16.6607, -11.9159) (-16.6549, -11.91) (-16.6491, -11.9042) (-16.6433, -11.8984) (-16.6376, -11.8926) (-16.6319, -11.8869) (-16.6263, -11.8812) (-16.6207, -11.8755) (-16.6152, -11.8698) (-16.6097, -11.8642) (-16.6043, -11.8586) (-16.5989, -11.853) (-16.5935, -11.8475) (-16.5882, -11.842) (-16.583, -11.8365) (-16.5778, -11.8311) (-16.5726, -11.8257) (-16.5675, -11.8203) (-16.5624, -11.8149) (-16.5574, -11.8096) (-16.5524, -11.8043) (-16.5475, -11.7991) (-16.5426, -11.7939) (-16.5378, -11.7887) (-16.533, -11.7835) (-16.5282, -11.7784) (-16.5236, -11.7733) (-16.5189, -11.7683) (-16.5143, -11.7633) (-16.5098, -11.7583) (-16.5053, -11.7534) (-16.5008, -11.7485) (-16.4964, -11.7436) (-16.492, -11.7388) (-16.4877, -11.734) (-16.4835, -11.7293) (-16.4793, -11.7246) (-16.4751, -11.7199) (-16.471, -11.7153) (-16.4669, -11.7107) (-16.4629, -11.7062) (-16.459, -11.7017) (-16.455, -11.6972) (-16.4512, -11.6928) (-16.4474, -11.6884) (-16.4436, -11.6841) (-16.4399, -11.6798) (-16.4362, -11.6755) (-16.4326, -11.6713) (-16.4291, -11.6672) (-16.4256, -11.6631) (-16.4221, -11.659) (-16.4187, -11.655) (-16.4153, -11.651) (-16.412, -11.6471) (-16.4088, -11.6432) (-16.4056, -11.6394) (-16.4024, -11.6356) (-16.3994, -11.6319) (-16.3963, -11.6283) (-16.3933, -11.6246) (-16.3904, -11.6211) (-16.3875, -11.6176) (-16.3847, -11.6141) (-16.3819, -11.6107) (-16.3792, -11.6073) (-16.3766, -11.604) (-16.374, -11.6008) (-16.3714, -11.5976) (-16.3689, -11.5945) (-16.3665, -11.5914) (-16.3641, -11.5884) (-16.3618, -11.5855) (-16.3595, -11.5826) (-16.3573, -11.5798) (-16.3551, -11.577) (-16.353, -11.5743) (-16.351, -11.5717) (-16.349, -11.5691) (-16.3471, -11.5666) (-16.3452, -11.5641) (-16.3434, -11.5618) (-16.3416, -11.5595) (-16.3399, -11.5572) (-16.3383, -11.5551) (-16.3367, -11.553) (-16.3352, -11.551) (-16.3338, -11.549) (-16.3324, -11.5471) (-16.331, -11.5453) (-16.3298, -11.5436) (-16.3286, -11.542) (-16.3274, -11.5404) (-16.3263, -11.5389) (-16.3253, -11.5375) (-16.3244, -11.5362) (-16.3235, -11.535) (-16.3227, -11.5338) (-16.3219, -11.5327) (-16.3212, -11.5317) (-16.3206, -11.5309) (-16.32, -11.5301) (-16.3195, -11.5294) (-16.3191, -11.5287) (-16.3188, -11.5283) (-16.3186, -11.5281) (-16.3185, -11.5279) (-16.3184, -11.5278) knots -1 -1 -1 -1 -1 -1 -0.99583333 -0.99166667 -0.9875 -0.98333333 -0.97916667 -0.975 -0.97083333 -0.96666667 -0.9625 -0.95833333 -0.95416667 -0.95 -0.94583333 -0.94166667 -0.9375 -0.93333333 -0.92916667 -0.925 -0.92083333 -0.91666667 -0.9125 -0.90833333 -0.90416667 -0.9 -0.89583333 -0.89166667 -0.8875 -0.88333333 -0.87916667 -0.875 -0.87083333 -0.86666667 -0.8625 -0.85833333 -0.85416667 -0.85 -0.84583333 -0.84166667 -0.8375 -0.83333333 -0.82916667 -0.825 -0.82083333 -0.81666667 -0.8125 -0.80833333 -0.80416667 -0.8 -0.79583333 -0.79166667 -0.7875 -0.78333333 -0.77916667 -0.775 -0.77083333 -0.76666667 -0.7625 -0.75833333 -0.75416667 -0.75 -0.74583333 -0.74166667 -0.7375 -0.73333333 -0.72916667 -0.725 -0.72083333 -0.71666667 -0.7125 -0.70833333 -0.70416667 -0.7 -0.69583333 -0.69166667 -0.6875 -0.68333333 -0.67916667 -0.675 -0.67083333 -0.66666667 -0.6625 -0.65833333 -0.65416667 -0.65 -0.64583333 -0.64166667 -0.6375 -0.63333333 -0.62916667 -0.625 -0.62083333 -0.61666667 -0.6125 -0.60833333 -0.60416667 -0.6 -0.59583333 -0.59166667 -0.5875 -0.58333333 -0.57916667 -0.575 -0.57083333 -0.56666667 -0.5625 -0.55833333 -0.55416667 -0.55 -0.54583333 -0.54166667 -0.5375 -0.53333333 -0.52916667 -0.525 -0.52083333 -0.51666667 -0.5125 -0.50833333 -0.50416667 -0.5 -0.49583333 -0.49166667 -0.4875 -0.48333333 -0.47916667 -0.475 -0.47083333 -0.46666667 -0.4625 -0.45833333 -0.45416667 -0.45 -0.44583333 -0.44166667 -0.4375 -0.43333333 -0.42916667 -0.425 -0.42083333 -0.41666667 -0.4125 -0.40833333 -0.40416667 -0.4 -0.39583333 -0.39166667 -0.3875 -0.38333333 -0.37916667 -0.375 -0.37083333 -0.36666667 -0.3625 -0.35833333 -0.35416667 -0.35 -0.34583333 -0.34166667 -0.3375 -0.33333333 -0.32916667 -0.325 -0.32083333 -0.31666667 -0.3125 -0.30833333 -0.30416667 -0.3 -0.29583333 -0.29166667 -0.2875 -0.28333333 -0.27916667 -0.275 -0.27083333 -0.26666667 -0.2625 -0.25833333 -0.25416667 -0.25 -0.24583333 -0.24166667 -0.2375 -0.23333333 -0.22916667 -0.225 -0.22083333 -0.21666667 -0.2125 -0.20833333 -0.20416667 -0.2 -0.19583333 -0.19166667 -0.1875 -0.18333333 -0.17916667 -0.175 -0.17083333 -0.16666667 -0.1625 -0.15833333 -0.15416667 -0.15 -0.14583333 -0.14166667 -0.1375 -0.13333333 -0.12916667 -0.125 -0.12083333 -0.11666667 -0.1125 -0.10833333 -0.10416667 -0.1 -0.09583333 -0.09166667 -0.0875 -0.08333333 -0.07916667 -0.075 -0.07083333 -0.06666667 -0.0625 -0.05833333 -0.05416667 -0.05 -0.04583333 -0.04166667 -0.0375 -0.03333333 -0.02916667 -0.025 -0.02083333 -0.01666667 -0.0125 -0.00833333 -0.00416667 0 0 0 0 0 0
  line L85 (-28.6734, 10.4033) -> (-28.9671, 10.3818)
  line L86 (-24.6806, -2.8132) -> (-24.6799, -2.8128)
  line L87 (-22.9441, -5.3086) -> (-22.7115, -5.1281)
  line L88 (-24.0271, -3.818) -> (-24.0278, -3.8184)
  line L89 (-22.1898, -6.2401) -> (-22.1904, -6.2406)
  arc A37 (-25.8803, -0.0209) -> (-25.3417, -1.078) centre (0, 12.5) ccw
  line L90 (-29.0298, 11.5787) -> (-28.7355, 11.5881)
  line L91 (-20.9575, -7.61) -> (-20.9569, -7.6094)
  line L92 (-20.9569, -7.6094) -> (-20.7445, -7.4055)
  line L93 (-23.7836, -3.6526) -> (-24.0271, -3.818)
  arc A38 (-24.4297, -2.6575) -> (-23.7836, -3.6526) centre (0, 12.5) ccw
  line L94 (-20.1094, -8.4569) -> (-20.11, -8.4575)
  arc A39 (-25.363, -5.3246) -> (-24.7898, -6.1136) centre (0, 12.5) ccw
  spline S27 degree 5 poles (-28.5147, 24.6618) (-28.5128, 24.66) (-28.5089, 24.6562) (-28.503, 24.6506) (-28.4951, 24.6432) (-28.4854, 24.634) (-28.4756, 24.6248) (-28.4658, 24.6156) (-28.4561, 24.6065) (-28.4464, 24.5973) (-28.4366, 24.5883) (-28.4269, 24.5792) (-28.4172, 24.5702) (-28.4075, 24.5613) (-28.3978, 24.5523) (-28.3882, 24.5434) (-28.3785, 24.5345) (-28.3689, 24.5257) (-28.3593, 24.5169) (-28.3496, 24.5081) (-28.34, 24.4994) (-28.3305, 24.4907) (-28.3209, 24.482) (-28.3113, 24.4734) (-28.3018, 24.4648) (-28.2922, 24.4562) (-28.2827, 24.4477) (-28.2732, 24.4392) (-28.2637, 24.4307) (-28.2542, 24.4223) (-28.2447, 24.4139) (-28.2353, 24.4055) (-28.2259, 24.3972) (-28.2164, 24.3889) (-28.207, 24.3807) (-28.1976, 24.3724) (-28.1882, 24.3643) (-28.1789, 24.3561) (-28.1695, 24.348) (-28.1602, 24.3399) (-28.1509, 24.3318) (-28.1416, 24.3238) (-28.1323, 24.3158) (-28.123, 24.3079) (-28.1137, 24.3) (-28.1045, 24.2921) (-28.0953, 24.2843) (-28.0861, 24.2765) (-28.0769, 24.2687) (-28.0677, 24.2609) (-28.0585, 24.2532) (-28.0494, 24.2456) (-28.0403, 24.2379) (-28.0312, 24.2303) (-28.0221, 24.2228) (-28.013, 24.2153) (-28.0039, 24.2078) (-27.9949, 24.2003) (-27.9859, 24.1929) (-27.9769, 24.1855) (-27.9679, 24.1781) (-27.9589, 24.1708) (-27.95, 24.1635) (-27.9411, 24.1563) (-27.9322, 24.1491) (-27.9233, 24.1419) (-27.9144, 24.1348) (-27.9055, 24.1276) (-27.8967, 24.1206) (-27.8879, 24.1135) (-27.8791, 24.1065) (-27.8704, 24.0996) (-27.8616, 24.0927) (-27.8529, 24.0858) (-27.8442, 24.0789) (-27.8355, 24.0721) (-27.8268, 24.0653) (-27.8182, 24.0585) (-27.8096, 24.0518) (-27.801, 24.0452) (-27.7924, 24.0385) (-27.7838, 24.0319) (-27.7753, 24.0253) (-27.7668, 24.0188) (-27.7583, 24.0123) (-27.7498, 24.0058) (-27.7414, 23.9994) (-27.733, 23.993) (-27.7246, 23.9867) (-27.7162, 23.9803) (-27.7078, 23.9741) (-27.6995, 23.9678) (-27.6912, 23.9616) (-27.6829, 23.9554) (-27.6747, 23.9493) (-27.6665, 23.9432) (-27.6582, 23.9371) (-27.6501, 23.9311) (-27.6419, 23.9251) (-27.6338, 23.9192) (-27.6257, 23.9132) (-27.6176, 23.9074) (-27.6096, 23.9015) (-27.6015, 23.8957) (-27.5936, 23.8899) (-27.5856, 23.8842) (-27.5776, 23.8785) (-27.5697, 23.8728) (-27.5618, 23.8672) (-27.554, 23.8616) (-27.5462, 23.8561) (-27.5384, 23.8506) (-27.5306, 23.8451) (-27.5228, 23.8396) (-27.5151, 23.8342) (-27.5074, 23.8289) (-27.4998, 23.8235) (-27.4922, 23.8183) (-27.4846, 23.813) (-27.477, 23.8078) (-27.4695, 23.8026) (-27.462, 23.7975) (-27.4545, 23.7924) (-27.447, 23.7873) (-27.4396, 23.7823) (-27.4323, 23.7773) (-27.4249, 23.7723) (-27.4176, 23.7674) (-27.4103, 23.7625) (-27.4031, 23.7577) (-27.3958, 23.7529) (-27.3887, 23.7481) (-27.3815, 23.7434) (-27.3744, 23.7387) (-27.3673, 23.734) (-27.3603, 23.7294) (-27.3533, 23.7248) (-27.3463, 23.7203) (-27.3393, 23.7158) (-27.3324, 23.7113) (-27.3256, 23.7069) (-27.3187, 23.7025) (-27.3119, 23.6982) (-27.3052, 23.6939) (-27.2985, 23.6896) (-27.2918, 23.6854) (-27.2851, 23.6812) (-27.2785, 23.677) (-27.272, 23.6729) (-27.2654, 23.6688) (-27.259, 23.6648) (-27.2525, 23.6608) (-27.2461, 23.6568) (-27.2397, 23.6529) (-27.2334, 23.649) (-27.2271, 23.6451) (-27.2209, 23.6413) (-27.2147, 23.6376) (-27.2085, 23.6338) (-27.2024, 23.6301) (-27.1963, 23.6265) (-27.1903, 23.6229) (-27.1843, 23.6193) (-27.1784, 23.6158) (-27.1725, 23.6123) (-27.1666, 23.6088) (-27.1608, 23.6054) (-27.155, 23.602) (-27.1493, 23.5987) (-27.1436, 23.5954) (-27.138, 23.5921) (-27.1324, 23.5889) (-27.1269, 23.5857) (-27.1214, 23.5826) (-27.116, 23.5795) (-27.1106, 23.5764) (-27.1053, 23.5734) (-27.1, 23.5704) (-27.0948, 23.5675) (-27.0896, 23.5646) (-27.0845, 23.5617) (-27.0794, 23.5589) (-27.0744, 23.5561) (-27.0694, 23.5534) (-27.0645, 23.5507) (-27.0597, 23.548) (-27.0549, 23.5454) (-27.0501, 23.5428) (-27.0454, 23.5403) (-27.0408, 23.5378) (-27.0362, 23.5353) (-27.0317, 23.5329) (-27.0272, 23.5306) (-27.0228, 23.5282) (-27.0185, 23.5259) (-27.0142, 23.5237) (-27.01, 23.5215) (-27.0058, 23.5193) (-27.0017, 23.5172) (-26.9977, 23.5151) (-26.9937, 23.5131) (-26.9898, 23.5111) (-26.986, 23.5091) (-26.9822, 23.5072) (-26.9785, 23.5053) (-26.9748, 23.5035) (-26.9713, 23.5017) (-26.9678, 23.4999) (-26.9643, 23.4982) (-26.961, 23.4966) (-26.9577, 23.4949) (-26.9544, 23.4934) (-26.9513, 23.4918) (-26.9482, 23.4903) (-26.9452, 23.4889) (-26.9423, 23.4875) (-26.9394, 23.4861) (-26.9366, 23.4848) (-26.9339, 23.4835) (-26.9313, 23.4823) (-26.9288, 23.4811) (-26.9263, 23.4799) (-26.924, 23.4788) (-26.9217, 23.4778) (-26.9195, 23.4768) (-26.9173, 23.4758) (-26.9153, 23.4749) (-26.9134, 23.474) (-26.9115, 23.4731) (-26.9097, 23.4724) (-26.908, 23.4716) (-26.9065, 23.4709) (-26.905, 23.4702) (-26.9036, 23.4696) (-26.9023, 23.4691) (-26.9011, 23.4685) (-26.9, 23.4681) (-26.899, 23.4676) (-26.8981, 23.4672) (-26.8973, 23.4669) (-26.8966, 23.4666) (-26.8961, 23.4664) (-26.8958, 23.4663) (-26.8956, 23.4662) (-26.8955, 23.4662) knots -1 -1 -1 -1 -1 -1 -0.99583333 -0.99166667 -0.9875 -0.98333333 -0.97916667 -0.975 -0.97083333 -0.96666667 -0.9625 -0.95833333 -0.95416667 -0.95 -0.94583333 -0.94166667 -0.9375 -0.93333333 -0.92916667 -0.925 -0.92083333 -0.91666667 -0.9125 -0.90833333 -0.90416667 -0.9 -0.89583333 -0.89166667 -0.8875 -0.88333333 -0.87916667 -0.875 -0.87083333 -0.86666667 -0.8625 -0.85833333 -0.85416667 -0.85 -0.84583333 -0.84166667 -0.8375 -0.83333333 -0.82916667 -0.825 -0.82083333 -0.81666667 -0.8125 -0.80833333 -0.80416667 -0.8 -0.79583333 -0.79166667 -0.7875 -0.78333333 -0.77916667 -0.775 -0.77083333 -0.76666667 -0.7625 -0.75833333 -0.75416667 -0.75 -0.74583333 -0.74166667 -0.7375 -0.73333333 -0.72916667 -0.725 -0.72083333 -0.71666667 -0.7125 -0.70833333 -0.70416667 -0.7 -0.69583333 -0.69166667 -0.6875 -0.68333333 -0.67916667 -0.675 -0.67083333 -0.66666667 -0.6625 -0.65833333 -0.65416667 -0.65 -0.64583333 -0.64166667 -0.6375 -0.63333333 -0.62916667 -0.625 -0.62083333 -0.61666667 -0.6125 -0.60833333 -0.60416667 -0.6 -0.59583333 -0.59166667 -0.5875 -0.58333333 -0.57916667 -0.575 -0.57083333 -0.56666667 -0.5625 -0.55833333 -0.55416667 -0.55 -0.54583333 -0.54166667 -0.5375 -0.53333333 -0.52916667 -0.525 -0.52083333 -0.51666667 -0.5125 -0.50833333 -0.50416667 -0.5 -0.49583333 -0.49166667 -0.4875 -0.48333333 -0.47916667 -0.475 -0.47083333 -0.46666667 -0.4625 -0.45833333 -0.45416667 -0.45 -0.44583333 -0.44166667 -0.4375 -0.43333333 -0.42916667 -0.425 -0.42083333 -0.41666667 -0.4125 -0.40833333 -0.40416667 -0.4 -0.39583333 -0.39166667 -0.3875 -0.38333333 -0.37916667 -0.375 -0.37083333 -0.36666667 -0.3625 -0.35833333 -0.35416667 -0.35 -0.34583333 -0.34166667 -0.3375 -0.33333333 -0.32916667 -0.325 -0.32083333 -0.31666667 -0.3125 -0.30833333 -0.30416667 -0.3 -0.29583333 -0.29166667 -0.2875 -0.28333333 -0.27916667 -0.275 -0.27083333 -0.26666667 -0.2625 -0.25833333 -0.25416667 -0.25 -0.24583333 -0.24166667 -0.2375 -0.23333333 -0.22916667 -0.225 -0.22083333 -0.21666667 -0.2125 -0.20833333 -0.20416667 -0.2 -0.19583333 -0.19166667 -0.1875 -0.18333333 -0.17916667 -0.175 -0.17083333 -0.16666667 -0.1625 -0.15833333 -0.15416667 -0.15 -0.14583333 -0.14166667 -0.1375 -0.13333333 -0.12916667 -0.125 -0.12083333 -0.11666667 -0.1125 -0.10833333 -0.10416667 -0.1 -0.09583333 -0.09166667 -0.0875 -0.08333333 -0.07916667 -0.075 -0.07083333 -0.06666667 -0.0625 -0.05833333 -0.05416667 -0.05 -0.04583333 -0.04166667 -0.0375 -0.03333333 -0.02916667 -0.025 -0.02083333 -0.01666667 -0.0125 -0.00833333 -0.00416667 0 0 0 0 0 0
  line L95 (-28.587, 7.3655) -> (-28.5878, 7.3654)